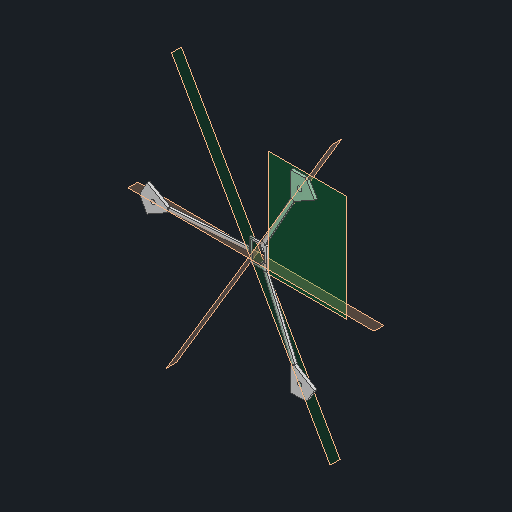
# Autodesk Inventor part: mpu_unit_holder
Saved by Autodesk Inventor 2024 (Build 280153000, 153)
## iProperties
Created: 2026-03-31
Part Number: mpu_unit_holder
Material: Generic
Document SubType Name: Modeling
Designer: schar
Density: 1 g/cm^3
Appearance: Default
Author: schar
Autodesk Inventor part; units mm, degrees
ref_plane "YZ Plane" through (0, 0, 0) normal (1, 0, 0) x (0, 1, 0)
ref_plane "XZ Plane" through (0, 0, 0) normal (0, 1, 0) x (-1, 0, 0)
ref_plane "XY Plane" through (0, 0, 0) normal (0, 0, 1) x (1, 0, 0)
sketch "Sketch1" plane through (0, 0, 0) normal (0, 0, 1) x (1, 0, 0)
  line L0 (-7.78, -10.1309) -> (7.78, -10.1309) projected
  line L1 (-7.78, 10.1309) -> (-7.78, -10.1309) projected
  line L2 (7.78, 10.1309) -> (-7.78, 10.1309) projected
  line L3 (7.78, -10.1309) -> (7.78, 10.1309) projected
  circle A0 centre (-6.3604, -8.6811) radius 0.9796 projected
  circle A1 centre (-6.411, 1.3369) radius 0.9537 projected
  circle A2 centre (-6.4264, 8.81) radius 1.0098 projected
  circle A3 centre (-6.4423, -1.2136) radius 0.9892 projected
  circle A4 centre (5.121, 7.4767) radius 1.5084 projected
  circle A5 centre (-6.3724, -6.2212) radius 0.9903 projected
  circle A6 centre (-6.3869, 3.7994) radius 0.9784 projected
  circle A7 centre (-6.4163, 6.3065) radius 0.9737 projected
  circle A8 centre (-6.3847, -3.6499) radius 0.9564 projected
  circle A9 centre (5.1439, -7.5842) radius 1.4324 projected
  circle A10 centre (5.121, 7.4767) radius 2.6542
  circle A11 centre (5.1439, -7.5842) radius 2.5467
  line L4 (5.121, 4.8225) -> (7.78, 4.8225)
  line L5 (2.4668, 7.4767) -> (2.4668, 10.1309)
  line L6 (5.1439, -5.0374) -> (7.78, -5.0374)
  line L7 (2.5971, -7.5842) -> (2.5971, -10.1309)
  line L8 (-9.78, 12.131) -> (9.78, 12.131)
  line L9 (9.78, 12.131) -> (9.78, -12.131)
  line L10 (9.78, -12.131) -> (-9.78, -12.131)
  line L11 (-9.78, -12.131) -> (-9.78, 12.131)
  line L12 (-9.78, 12.131) -> (9.78, -12.131) construction
  line L13 (9.78, 12.131) -> (-9.78, -12.131) construction
  point P0 (0, 0)
  dimension "d0" = 19.56
  dimension "d1" = 24.262
  constraints: 20 end point, 6 tangent, 5 perpendicular, 4 point on circle, 4 point on line, 2 centre point, 2 coincident, 2 midpoint, 2 parallel, 1 horizontal
  measures "d0" distance of L9.end L10.end
  measures "d1" distance of L8.end L9.end
extrude "Extrusion1" add sketch "Sketch1" along normal blind 2 contours L7 A11 L0 | A11 L6 L3 L0 | A11 | L2 A10 L5 | L2 L3 L4 A10 | A10 | L8 L9 L10 L11
ref_plane "Work Plane1" through (50.8312, 84.4361, 10) normal (0, 0, -1) x (1, -0.0000013, 0)
sketch "Sketch2" plane through (50.8312, 84.4361, 10) normal (0, 0, -1) x (1, -0.0000013, 0)
  circle A0 centre (12.9878, 6.3432) radius 1.5 projected
  circle A1 centre (-16.5452, -10.0614) radius 1.5 projected
  line L0 (29.2785, 8.2439) -> (6.972, 21.6013) projected
  line L1 (6.972, 21.6013) -> (-2.5648, 5.6752) projected
  line L2 (-2.5648, 5.6752) -> (-6.7072, 3.2563) projected
  line L3 (-6.7072, 3.2563) -> (-26.7047, 2.9374) projected
  line L4 (-26.7047, 2.9374) -> (-26.7047, -0.0626) projected
  line L5 (-26.7047, -0.0626) -> (-26.3857, -20.0601) projected
  line L6 (-26.3857, -20.0601) -> (-26.3857, -23.0601) projected
  line L7 (-26.3857, -23.0601) -> (9.051, -22.741) projected
  line L8 (9.051, -22.741) -> (11.5978, -21.2824) projected
  line L9 (11.5978, -21.2824) -> (29.2785, 8.2439) projected
  circle A2 centre (3.451, -9.5829) radius 2.5 projected
  circle A3 centre (-15.11, 178.7515) radius 1.5 projected
  circle A4 centre (13.8632, 161.3775) radius 1.5 projected
  line L10 (-24.9015, 191.9093) -> (-25.316, 165.9126) projected
  line L11 (-25.316, 165.9126) -> (-6.7552, 165.6166) projected
  line L12 (-6.7552, 165.6166) -> (-2.5892, 163.2386) projected
  line L13 (-2.5892, 163.2386) -> (7.6858, 146.0798) projected
  line L14 (7.6858, 146.0798) -> (10.2838, 147.5798) projected
  line L15 (10.2838, 147.5798) -> (27.4427, 157.8548) projected
  line L16 (27.4427, 157.8548) -> (30.0407, 159.3548) projected
  line L17 (30.0407, 159.3548) -> (12.0461, 189.8843) projected
  line L18 (12.0461, 189.8843) -> (9.5094, 191.3606) projected
  line L19 (9.5094, 191.3606) -> (-24.9015, 191.9093) projected
  circle A5 centre (3.4508, 178.4555) radius 2.5 projected
  circle A6 centre (-150.371, 68.2138) radius 1.5 projected
  circle A7 centre (-149.8114, 101.9924) radius 1.5 projected
  line L20 (-156.8703, 53.1553) -> (-134.1492, 65.7946) projected
  line L21 (-134.1492, 65.7946) -> (-143.1733, 82.0168) projected
  line L22 (-143.1733, 82.0168) -> (-143.1969, 86.8137) projected
  line L23 (-143.1969, 86.8137) -> (-133.4744, 104.2915) projected
  line L24 (-133.4744, 104.2915) -> (-136.0725, 105.7915) projected
  line L25 (-136.0725, 105.7915) -> (-153.5503, 115.5139) projected
  line L26 (-153.5503, 115.5139) -> (-156.1484, 117.0139) projected
  line L27 (-156.1484, 117.0139) -> (-173.5903, 86.1653) projected
  line L28 (-173.5903, 86.1653) -> (-173.6005, 83.2304) projected
  line L29 (-173.6005, 83.2304) -> (-156.8703, 53.1553) projected
  circle A8 centre (-159.3951, 84.436) radius 2.5 projected
  line L30 (-6.7072, 3.2563) -> (-6.2903, -22.8792)
  line L31 (-2.5648, 5.6752) -> (20.1679, -6.9705)
  line L32 (-2.5892, 163.2386) -> (19.8363, 176.6674)
  line L33 (-6.7552, 165.6166) -> (-6.3406, 191.6133)
  line L34 (-143.1969, 86.8137) -> (-166.0393, 99.5203)
  line L35 (-143.1733, 82.0168) -> (-165.8944, 69.3775)
  line L36 (-149.8114, 101.9924) -> (-154.6181, 93.167)
  line L37 (-150.371, 68.2138) -> (-154.5338, 75.6971)
  line L38 (13.8632, 161.3775) -> (8.6236, 169.953)
  line L39 (-15.11, 178.7515) -> (-6.5479, 178.615)
  line L40 (12.9878, 6.3432) -> (8.8016, -0.6476)
  line L41 (-16.5452, -10.0614) -> (-6.4948, -10.0614)
  line L42 (-41.0511, 72.3051) -> (-60.6111, 72.3052) projected
  line L43 (-60.6111, 72.3052) -> (-60.6111, 96.5672) projected
  line L44 (-2.549, 143.4361) -> (-2.5491, 94.4361) projected
  line L45 (-60.6111, 96.5672) -> (-41.0511, 96.5671) projected
  line L46 (-41.0511, 96.5671) -> (-41.0511, 72.3051) projected
  circle A9 centre (-45.7101, 76.9595) radius 1.5084 projected
  circle A10 centre (-45.6872, 92.0203) radius 1.4324 projected
  line L47 (-6.5479, 178.615) -> (8.6236, 169.953)
  line L48 (8.6236, 169.953) -> (-120.1954, -55.6742)
  line L49 (-6.5479, 178.615) -> (-103.8184, 8.2451)
  line L50 (-6.4948, -10.0614) -> (8.6236, -0.5486)
  line L51 (-6.4948, -10.0614) -> (-92.7123, 126.962)
  line L52 (8.6236, -0.5486) -> (-96.6324, 166.7321)
  line L53 (-154.5338, 93.1201) -> (-154.5338, 75.6971)
  line L54 (-154.5338, 75.6971) -> (9.5512, 75.6971)
  line L55 (-154.5338, 93.1201) -> (4.4207, 93.1201)
  point P0 (-50.8311, 84.4361)
  dimension "d4" = 61.19
  dimension "d5" = 118.735
  constraints: 42 end point, 12 perpendicular, 9 point on line, 6 midpoint, 1 horizontal, 1 parallel, 1 vertical
  measures "d4" angle of L47 L33
  measures "d5" angle of L50 L31
extrude "Extrusion2" add sketch "Sketch2" along normal blind 3 contours L9 L8 L7 L30 L50 L31 | L31 L50 L30 L2 | L12 L33 L47 L32 | L47 L33 L19 L18 L17 L32 | L22 L35 L53 L34 | L53 L35 L29 L28 L27 L34
ref_plane "Work Plane2" through (54.2818, -94.0194, 10) normal (-0.8684276, -0.4958161, 0) x (-0.4958161, 0.8684276, 0)
ref_plane "Work Plane3" through (54.2822, 94.019, 10) normal (0.8578983, -0.5138195, 0) x (-0.5138195, -0.8578983, 0)
ref_plane "Work Plane4" through (-108.564, 0.0003, 10) normal (0.0048253, 0.9999884, 0) x (0.9999884, -0.0048253, 0)
sketch "Sketch4" plane through (54.2822, 94.019, 10) normal (0.8578983, -0.5138195, 0) x (-0.5138195, -0.8578983, 0)
  line L0 (4.9164, 0) -> (164.3854, 0) projected
  line L1 (8.7629, 0) -> (4.9164, 0) projected
  line L2 (166.5924, 0) -> (87.703, 0) projected
  line L3 (103.168, 8) -> (123.9823, 8) projected
  line L4 (-6.3482, 0) -> (16.1809, 0) projected
  line L5 (16.1809, 0) -> (16.1809, 3) projected
  line L6 (-6.3482, 3) -> (16.1809, 3) projected
  line L7 (-6.3482, 0) -> (-6.3482, 3) projected
  line L8 (113.932, 10) -> (93.1177, 10) projected
  line L9 (4.9164, 3) -> (93.1177, 10)
  line L10 (93.1177, 10) -> (93.2764, 8)
  line L11 (93.2764, 8) -> (4.9164, 0)
  point P0 (108.55, 10)
  point P1 (6805.2142, -38858.9067)
  point P2 (16.1809, 1.0199)
  constraints: 6 end point, 1 midpoint, 1 perpendicular
extrude "Extrusion3" add sketch "Sketch4" along normal mid plane 4 contours L5 L6 L9 L10 L11
sketch "Sketch5" plane through (-108.564, 0.0003, 10) normal (0.0048253, 0.9999884, 0) x (0.9999884, -0.0048253, 0)
  line L0 (-6.5718, 0) -> (16.21, 0) projected
  line L1 (16.21, 0) -> (16.21, 3) projected
  line L2 (-6.5718, 3) -> (16.21, 3) projected
  line L3 (-6.5718, 0) -> (-6.5718, 3) projected
  line L4 (98.8414, 10) -> (118.4011, 10) projected
  line L5 (98.8414, 10) -> (4.8191, 3)
  line L6 (-6.5718, 0) -> (16.21, 0) projected
  line L7 (98.8414, 8) -> (118.4011, 8) projected
  line L8 (4.8191, 0) -> (98.8414, 8)
  line L9 (4.8191, 3) -> (4.8191, 0)
  line L10 (98.8414, 10) -> (98.8414, 8)
  point P0 (108.5627, 10)
  point P1 (16.21, 0.9692)
  constraints: 8 end point, 2 midpoint, 1 perpendicular, 1 vertical
extrude "Extrusion4" add sketch "Sketch5" along normal mid plane 4 contours L1 L2 L5 L10 L8
sketch "Sketch6" plane through (54.2818, -94.0194, 10) normal (-0.8684276, -0.4958161, 0) x (-0.4958161, 0.8684276, 0)
  line L0 (-6.5718, 0) -> (16.21, 0) projected
  line L1 (16.21, 0) -> (16.21, 3) projected
  line L2 (-6.5718, 3) -> (16.21, 3) projected
  line L3 (-6.5718, 0) -> (-6.5718, 3) projected
  line L4 (102.877, 10) -> (93.1789, 10) projected
  line L5 (4.8191, 3) -> (93.1789, 10)
  line L6 (102.877, 8) -> (93.1789, 8) projected
  line L7 (93.1789, 10) -> (93.1789, 8)
  line L8 (93.1789, 8) -> (4.8191, 0)
  line L9 (4.8191, 3) -> (4.8191, 0)
  point P0 (108.5629, 10)
  constraints: 8 end point, 2 midpoint, 1 perpendicular, 1 vertical
extrude "Extrusion5" add sketch "Sketch6" along normal mid plane 4 contours L9 L2 L1 L8 | L1 L2 L5 L7 L8
sketch "Sketch7" plane through (0, 0, 0) normal (0, 0, -1) x (-1, 0, 0)
  line L0 (9.78, -12.131) -> (-9.78, -12.131) projected
  line L1 (9.78, 12.131) -> (9.78, -12.131) projected
  line L2 (-9.78, 12.131) -> (9.78, 12.131) projected
  line L3 (-9.78, -12.131) -> (-9.78, 12.131) projected
  circle A0 centre (-5.121, 7.4767) radius 1.5084 projected
  circle A1 centre (-5.1439, -7.5842) radius 1.4324 projected
  arc A2 (-2.5971, -7.5842) -> (-5.1439, -5.0374) centre (-5.1439, -7.5842) ccw projected
  line L4 (-7.78, -5.0374) -> (-5.1439, -5.0374) projected
  line L5 (-7.78, 4.8225) -> (-7.78, -5.0374) projected
  line L6 (-5.121, 4.8225) -> (-7.78, 4.8225) projected
  arc A3 (-5.121, 4.8225) -> (-2.4668, 7.4767) centre (-5.121, 7.4767) ccw projected
  line L7 (-2.4668, 10.1309) -> (-2.4668, 7.4767) projected
  line L8 (7.78, 10.1309) -> (-2.4668, 10.1309) projected
  line L9 (7.78, -10.1309) -> (7.78, 10.1309) projected
  line L10 (-2.5971, -10.1309) -> (7.78, -10.1309) projected
  line L11 (-2.5971, -7.5842) -> (-2.5971, -10.1309) projected
  line L12 (-50.0403, 90.8289) -> (-4.7207, 15.1611) projected
  line L13 (-4.7207, 15.1611) -> (-2.9059, 12.131)
  line L14 (-8.1523, 13.1059) -> (-53.4719, 88.7736) projected
  line L15 (-8.1523, 13.1059) -> (-7.5685, 12.131)
  line L16 (-44.5078, -80.9339) -> (-6.3454, -14.092) projected
  line L17 (-6.3454, -14.092) -> (-5.2258, -12.131)
  line L18 (-8.1523, 13.1059) -> (-4.7207, 15.1611) projected
  line L19 (-6.3454, -14.092) -> (-9.78, -12.131) projected
  point P0 (0, 0)
  constraints: 6 end point, 3 collinear, 3 point on line
extrude "Extrusion6" add sketch "Sketch7" against normal blind 2 contours L17 L19 L0 | L2 L15 L18 L13
body "Solid1"
